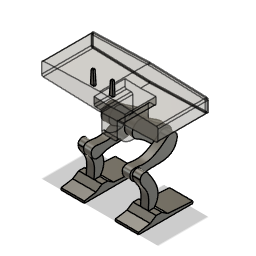
Mech v3 (Autodesk Fusion 360 design; units mm, degrees)
Autodesk Fusion 360 part; units mm, degrees
sketch "Esquisse1" plane through (0, 0, 0) normal (0, 0, 1) x (1, 0, 0)
  line L0 (-150, 33.8689) -> (-150, 61.1311)
  line L1 (-146.1333, 65.1289) -> (0, 70)
  line L2 (-146.1333, 29.8711) -> (0, 25)
  line L3 (146.1333, 65.1289) -> (0, 70)
  line L4 (150, 33.8689) -> (150, 61.1311)
  line L5 (146.1333, 29.8711) -> (0, 25)
  arc A0 (-146.1333, 65.1289) -> (-150, 61.1311) centre (-146, 61.1311) ccw
  arc A1 (-150, 33.8689) -> (-146.1333, 29.8711) centre (-146, 33.8689) ccw
  arc A2 (150, 61.1311) -> (146.1333, 65.1289) centre (146, 61.1311) ccw
  arc A3 (146.1333, 29.8711) -> (150, 33.8689) centre (146, 33.8689) ccw
  line L6 (146.0333, 62.1306) -> (0, 66.9983)
  line L7 (-146.0333, 62.1306) -> (0, 66.9983)
  arc A4 (-146.0333, 62.1306) -> (-147, 61.1311) centre (-146, 61.1311) ccw
  line L8 (-147, 33.8689) -> (-147, 61.1311)
  arc A5 (-147, 33.8689) -> (-146.0333, 32.8694) centre (-146, 33.8689) ccw
  line L9 (-146.0333, 32.8694) -> (0, 28.0017)
  line L10 (146.0333, 32.8694) -> (0, 28.0017)
  arc A6 (146.0333, 32.8694) -> (147, 33.8689) centre (146, 33.8689) ccw
  line L11 (147, 33.8689) -> (147, 61.1311)
  arc A7 (147, 61.1311) -> (146.0333, 62.1306) centre (146, 61.1311) ccw
  dimension "d3" = 4
  dimension "d4" = 4
  dimension "d5" = 4
  dimension "d6" = 4
  dimension "d7" = -3
  constraint tangent L0 A0
  constraint tangent L1 A0
  constraint tangent L2 A1
  constraint tangent L0 A1
  constraint tangent L3 A2
  constraint tangent L4 A2
  constraint tangent L5 A3
  constraint tangent L4 A3
  measures "d3" radius of A0
  measures "d4" radius of A1
  measures "d5" radius of A2
  measures "d6" radius of A3
extrude "Extrusion1" add sketch "Esquisse1" along normal blind 130 contours L0 L1 L2 L3 L4 L5 A0 A1 A2 A3 | L6 L7 A4 L8 A5 L9 L10 A6 L11 A7 makes body 1
extrude "Extrusion2" cut sketch "Esquisse1" along normal blind 5 contours L6 L7 A4 L8 A5 L9 L10 A6 L11 A7 bodies 1
move_body "Déplacer1" bodies 1 to x (1, 0, 0) y (0, 1, 0) z (0, 0, 1) at (0, 200, 0)
ref_plane "Plan de construction1" through (0, 225, 65) normal (0, 1, 0) x (0, 0, 1)
sketch "Esquisse2" plane through (0, 225, 0) normal (0, 1, 0) x (1, 0, 0)
  line L0 (40, -105) -> (-40, -105)
  line L1 (-40, -105) -> (-40, -25)
  line L2 (-40, -25) -> (40, -25)
  line L3 (40, -25) -> (40, -105)
  line L4 (146.1333, 0) -> (0, 0)
  dimension "d13" = 25
  constraint horizontal L0
  constraint vertical L1
  constraint horizontal L2
  constraint vertical L3
  measures "d13" distance of L2 L4
extrude "Extrusion3" cut sketch "Esquisse2" along normal blind 5 bodies 1
sketch "Esquisse3" plane through (0, 0, 105) normal (0, 0, -1) x (-1, 0, 0)
  line L0 (0, 225) -> (40, 226.3333)
  line L1 (40, 226.3333) -> (40, 230)
  line L2 (40, 230) -> (-40, 230)
  line L3 (-40, 230) -> (-40, 226.3333)
  line L4 (-40, 226.3333) -> (0, 225)
  line L5 (-40, 230) -> (40, 230)
  line L6 (40, 230) -> (40, 209)
  line L7 (36, 205) -> (24, 205)
  line L8 (20, 201) -> (20, 159)
  line L9 (16, 155) -> (-16, 155)
  line L10 (-20, 159) -> (-20, 201)
  line L11 (-24, 205) -> (-36, 205)
  line L12 (-40, 209) -> (-40, 230)
  arc A0 (-40, 209) -> (-36, 205) centre (-36, 209) ccw
  arc A1 (-20, 201) -> (-24, 205) centre (-24, 201) ccw
  arc A2 (-20, 159) -> (-16, 155) centre (-16, 159) ccw
  arc A3 (16, 155) -> (20, 159) centre (16, 159) ccw
  arc A4 (24, 205) -> (20, 201) centre (24, 201) ccw
  arc A5 (36, 205) -> (40, 209) centre (36, 209) ccw
  point P0 (20, 205)
  point P1 (20, 155)
  dimension "d16" = 50
  dimension "d17" = 4
  dimension "d18" = 4
  dimension "d19" = 4
  dimension "d20" = 4
  dimension "d21" = 4
  dimension "d22" = 4
  constraint coincident L2.end L3.start
  constraint coincident L1.end L2.start
  constraint perpendicular L5 L6
  constraint perpendicular L6 L7
  constraint perpendicular L7 L8
  constraint perpendicular L8 L9
  constraint perpendicular L9 L10
  constraint perpendicular L10 L11
  constraint perpendicular L5 L12
  constraint tangent L11 A0
  constraint tangent L12 A0
  constraint tangent L10 A1
  constraint tangent L11 A1
  constraint tangent L9 A2
  constraint tangent L10 A2
  constraint coincident P1 L9
  constraint coincident P1 L8
  constraint tangent L9 A3
  constraint tangent L8 A3
  constraint coincident P0 L8
  constraint coincident P0 L7
  constraint tangent L8 A4
  constraint tangent L7 A4
  constraint tangent L7 A5
  constraint tangent L6 A5
  measures "d16" distance of P0 P1
  measures "d17" radius of A0
  measures "d18" radius of A1
  measures "d19" radius of A2
  measures "d20" radius of A3
  measures "d21" radius of A4
  measures "d22" radius of A5
extrude "Extrusion4" add sketch "Esquisse3" along normal blind 80 bodies 1
sketch "Esquisse4" plane through (-20, 0, 0) normal (-1, 0, 0) x (0, 0, 1)
  line L0 (105, 159) -> (105, 201)
  line L1 (105, 201) -> (25, 201)
  line L2 (25, 201) -> (25, 159)
  line L3 (25, 159) -> (105, 159)
  line L4 (65, 205) -> (65, 155) construction
  line L5 (65, 155) -> (65, 205) construction
  arc A0 (25, 180) -> (105, 180) centre (65, 180) ccw
  line L6 (25, 180) -> (105, 180)
  dimension "d25" = 80
  constraint perpendicular L3 L4
  constraint midpoint L5 A0.centre
  constraint coincident L2 A0.start
  constraint coincident L0 A0.end
  constraint perpendicular L0 L6
  measures "d25" diameter of A0
extrude "Extrusion5" add sketch "Esquisse4" against normal blind 40 contours L3 A0 L6 | L3 A0 bodies 1
sketch "Esquisse5" plane through (-20, 0, 0) normal (-1, 0, 0) x (0, 0, 1)
  line L0 (25, 201) -> (25, 159)
  line L1 (25, 159) -> (30.9559, 159)
  arc A0 (30.9559, 159) -> (99.0441, 159) centre (65, 180) ccw
  line L2 (99.0441, 159) -> (105, 159)
  line L3 (105, 159) -> (105, 201)
  line L4 (105, 201) -> (25, 201)
  spline S0 degree 5 poles (50, 190) (48.5943, 188.5173) (45.7562, 185.6074) (41.4185, 181.4094) (35.4733, 176.1465) (27.7946, 170.1152) (19.9379, 164.5925) (12.0468, 159.4932) (4.3635, 154.6691) (-2.741, 149.8879) (-8.7472, 144.8223) (-13.1055, 139.1738) (-15.3557, 132.8001) (-15.2312, 125.8208) (-12.8105, 118.7889) (-8.4782, 112.5876) (-2.7614, 108.1375) (3.7842, 106.1866) (10.7306, 107.0074) (17.8284, 110.3413) (24.9477, 115.6146) (32.0463, 122.0851) (39.131, 129.0014) (46.216, 135.7855) (53.3085, 142.0733) (60.4134, 147.6486) (66.109, 151.4582) (70.3875, 153.9361) (73.2429, 155.4199) (74.6713, 156.1197) knots 0 0 0 0 0 0 0.04 0.08 0.12 0.16 0.2 0.24 0.28 0.32 0.36 0.4 0.44 0.48 0.52 0.56 0.6 0.64 0.68 0.72 0.76 0.8 0.84 0.88 0.92 0.96 1 1 1 1 1 1
  arc A1 (74.131, 155.8526) -> (49.3011, 189.2669) centre (65, 175) ccw
  point P0 (5, 155)
  point P1 (-15, 130)
  point P2 (0.8234, 107.4241)
  point P3 (35, 125)
  constraint coincident S0.start A1
  constraint coincident S0.end A1
  constraint coincident S0 A1.end
  constraint coincident S0 A1.start
extrude "Extrusion6" add sketch "Esquisse5" along normal blind 20 separate body contours L0 L1 A0 S0 A1 | L0 L1 A0 S0 makes body 2
sketch "Esquisse6" plane through (-40, 0, 0) normal (-1, 0, 0) x (0, 0, 1)
  spline S0 degree 5 poles (74.131, 155.8526) (74.2391, 155.9065) (74.3471, 155.9601) (74.4552, 156.0136) (74.5633, 156.0668) (74.6713, 156.1197) knots 0.996974 0.996974 0.996974 0.996974 0.996974 0.996974 1 1 1 1 1 1
  arc A0 (74.6713, 156.1197) -> (50, 190) centre (65, 175) ccw
  spline S1 degree 5 poles (50, 190) (49.8605, 189.8528) (49.7208, 189.7059) (49.5811, 189.5593) (49.4412, 189.413) (49.3011, 189.2669) knots 0 0 0 0 0 0 0.00397 0.00397 0.00397 0.00397 0.00397 0.00397
  spline S2 degree 5 poles (49.3011, 189.2669) (48.0302, 187.9413) (45.3253, 185.1916) (41.1233, 181.1485) (35.3209, 176.0267) (27.7946, 170.1152) (19.9379, 164.5925) (12.0468, 159.4932) (4.3635, 154.6691) (-2.741, 149.8879) (-8.7472, 144.8223) (-13.1055, 139.1738) (-15.3557, 132.8001) (-15.2312, 125.8208) (-12.8105, 118.7889) (-8.4782, 112.5876) (-2.7614, 108.1375) (3.7842, 106.1866) (10.7306, 107.0074) (17.8284, 110.3413) (24.9477, 115.6146) (32.0463, 122.0851) (39.131, 129.0014) (46.216, 135.7855) (53.3085, 142.0733) (60.3059, 147.5642) (65.8935, 151.3139) (70.0638, 153.7479) (72.8109, 155.1939) (74.131, 155.8526) knots 0.00397 0.00397 0.00397 0.00397 0.00397 0.00397 0.04 0.08 0.12 0.16 0.2 0.24 0.28 0.32 0.36 0.4 0.44 0.48 0.52 0.56 0.6 0.64 0.68 0.72 0.76 0.8 0.84 0.88 0.92 0.96 0.996974 0.996974 0.996974 0.996974 0.996974 0.996974
  spline S3 degree 5 poles (-8.5063, 123.5236) (-8.1226, 121.791) (-7.2435, 118.4579) (-5.5903, 113.854) (-2.7158, 108.5079) (1.9828, 103.1375) (7.7462, 99.0459) (14.4865, 96.1594) (22.0545, 94.3508) (30.2168, 93.4202) (38.6554, 93.0927) (47.0224, 93.0622) (54.9848, 93.0257) (62.2732, 92.7217) (68.7283, 91.9664) (74.3503, 90.6921) (79.3449, 88.984) (84.0154, 87.0599) (88.6532, 85.2541) (93.439, 83.9929) (98.3134, 83.7935) (103.0122, 85.1344) (107.1615, 88.274) (110.3514, 93.094) (112.2218, 98.9085) (112.4972, 104.726) (111.0241, 109.5548) (107.8019, 112.6688) (103.0306, 113.9507) (97.0589, 113.7856) (90.3019, 112.823) (83.1723, 111.7929) (75.9995, 111.2806) (68.9759, 111.5793) (62.1958, 112.7798) (55.6779, 114.8205) (49.3948, 117.5544) (43.2975, 120.8045) (37.3462, 124.4325) (31.5155, 128.3494) (25.7893, 132.4999) (21.2856, 135.9852) (17.95, 138.6875) (15.745, 140.5283) (14.6471, 141.4585) knots 0 0 0 0 0 0 0.025 0.05 0.075 0.1 0.125 0.15 0.175 0.2 0.225 0.25 0.275 0.3 0.325 0.35 0.375 0.4 0.425 0.45 0.475 0.5 0.525 0.55 0.575 0.6 0.625 0.65 0.675 0.7 0.725 0.75 0.775 0.8 0.825 0.85 0.875 0.9 0.925 0.95 0.975 1 1 1 1 1 1
  arc A1 (14.7156, 141.4005) -> (-8.5063, 123.5236) centre (5, 130) ccw
  point P0 (20, 95)
  point P1 (68.4132, 91.856)
  point P2 (90, 85)
  point P3 (107.1929, 88.9905)
  point P4 (110, 110)
  point P5 (84.842, 112.1055)
  point P6 (47.5906, 118.6006)
  constraint coincident S3.end A1
  constraint coincident S3 A1.start
extrude "Extrusion7" add sketch "Esquisse6" along normal blind 20 contours S2 S3 | S2 S3 A1 bodies 2
sketch "Esquisse7" plane through (-60, 0, 0) normal (-1, 0, 0) x (0, 0, 1)
  line L0 (14.7156, 141.4005) -> (14.6471, 141.4585)
  arc A0 (14.6471, 141.4585) -> (-8.5063, 123.5236) centre (5, 130) ccw
  spline S0 degree 5 poles (-8.5063, 123.5236) (-8.1226, 121.791) (-7.2435, 118.4579) (-5.5903, 113.854) (-2.7158, 108.5079) (1.9828, 103.1375) (7.7462, 99.0459) (14.4865, 96.1594) (22.0545, 94.3508) (30.2168, 93.4202) (38.6554, 93.0927) (47.0224, 93.0622) (54.9848, 93.0257) (62.2732, 92.7217) (68.7283, 91.9664) (74.3503, 90.6921) (79.3449, 88.984) (84.0154, 87.0599) (88.6532, 85.2541) (93.439, 83.9929) (98.3134, 83.7935) (103.0122, 85.1344) (107.1615, 88.274) (110.3514, 93.094) (112.2218, 98.9085) (112.4972, 104.726) (111.0241, 109.5548) (107.8019, 112.6688) (103.0306, 113.9507) (97.0589, 113.7856) (90.3019, 112.823) (83.1723, 111.7929) (75.9995, 111.2806) (68.9759, 111.5793) (62.1958, 112.7798) (55.6779, 114.8205) (49.3948, 117.5544) (43.2975, 120.8045) (37.3462, 124.4325) (31.5155, 128.3494) (25.8036, 132.4895) (21.3137, 135.9634) (17.9916, 138.6538) (15.7999, 140.4824) (14.7156, 141.4005) knots 0 0 0 0 0 0 0.025 0.05 0.075 0.1 0.125 0.15 0.175 0.2 0.225 0.25 0.275 0.3 0.325 0.35 0.375 0.4 0.425 0.45 0.475 0.5 0.525 0.55 0.575 0.6 0.625 0.65 0.675 0.7 0.725 0.75 0.775 0.8 0.825 0.85 0.875 0.9 0.925 0.95 0.975 0.999688 0.999688 0.999688 0.999688 0.999688 0.999688
  spline S1 degree 5 poles (84.4841, 103.2274) (83.0085, 101.166) (80.154, 97.0756) (76.1623, 91.0374) (71.4299, 83.1848) (66.5704, 73.724) (62.8807, 64.6564) (60.4933, 56.0265) (59.5296, 47.8752) (60.0385, 40.2189) (61.9589, 33.037) (64.5542, 27.6473) (67.0622, 23.7939) (68.9798, 21.3075) (70, 20.0849) knots 0 0 0 0 0 0 0.1 0.2 0.3 0.4 0.5 0.6 0.7 0.8 0.9 1 1 1 1 1 1
  spline S2 degree 5 poles (106, 100) (106, 98.7107) (105.838, 96.1843) (105.1087, 92.5515) (103.2345, 87.99) (99.8024, 82.5801) (95.8269, 77.2362) (91.8872, 71.7356) (88.4972, 65.9101) (86.0067, 59.6978) (84.4968, 53.1998) (83.856, 46.6287) (83.8501, 40.2612) (84.1893, 34.3904) (84.5883, 29.2814) (84.8343, 25.1174) (84.8325, 22.5956) (84.7064, 21.1632) (84.5674, 20.4106) (84.4841, 20.0849) knots 0 0 0 0 0 0 0.066667 0.133333 0.2 0.266667 0.333333 0.4 0.466667 0.533333 0.6 0.666667 0.733333 0.8 0.866667 0.933333 1 1 1 1 1 1
  line L1 (70, 20.0849) -> (55, 10)
  line L2 (100, 10) -> (84.4841, 20.0849)
  line L3 (55, 10) -> (-10, 5)
  line L4 (-10, 5) -> (-10, 0)
  line L5 (-10, 0) -> (130, 0)
  line L6 (130, 0) -> (130, 5)
  line L7 (130, 5) -> (100, 10)
  arc A1 (106, 100) -> (84.4841, 103.2274) centre (95, 100) ccw
  line L8 (70, 20.0849) -> (84.4841, 20.0849)
  point P0 (60, 50)
  point P1 (88.7009, 65.7756)
  point P2 (84.4841, 30.4969)
  dimension "d32" = 22
  constraint tangent S2 A1
  constraint perpendicular L4 L5
  constraint horizontal L8
  measures "d32" diameter of A1
extrude "Extrusion8" add sketch "Esquisse7" along normal blind 20 contours S0 S1 S2 L8 | S0 S1 S2 A1 bodies 2
extrude "Extrusion9" add sketch "Esquisse7" along normal blind 40 and the other way blind 20 contours L1 L2 L3 L4 L5 L6 L7 L8 bodies 2
mirror "Symétrie miroir1" about plane through (0, 0, 0) normal (1, 0, 0) of bodies 2 makes body 3
ref_plane "Plan de construction2" through (0, 247.5, 125) normal (0, 0, 1) x (1, 0, 0)
sketch "Esquisse8" plane through (0, 0, 125) normal (0, 0, 1) x (1, 0, 0)
  line L0 (-25, 269) -> (-19.7782, 269)
  line L1 (-19.7782, 269) -> (-22.3891, 304.2057)
  line L2 (-22.3891, 304.2057) -> (-27.3754, 303.8359)
  line L3 (-27.3754, 303.8359) -> (-29, 269)
  line L4 (-29, 269) -> (-25, 269)
  line L5 (0, 314) -> (0, 260) construction
  line L6 (22.3891, 304.2057) -> (27.3754, 303.8359)
  line L7 (27.3754, 303.8359) -> (29, 269)
  line L8 (19.7782, 269) -> (22.3891, 304.2057)
  line L9 (25, 269) -> (19.7782, 269)
  line L10 (29, 269) -> (25, 269)
  dimension "d42" = 5
  constraint horizontal L0
  constraint perpendicular L1 L2
  constraint parallel L0 L4
  constraint symmetric L0.start L5 L9.start
  constraint symmetric L0.end L5 L8.start
  constraint symmetric L1.end L5 L6.start
  constraint symmetric L2.end L5 L6.end
  constraint symmetric L3.end L5 L7.end
  measures "d42" distance of L1.end L2.end
extrude "Extrusion10" add sketch "Esquisse8" against normal blind 5 separate body makes body 4 at (25.3845, 280.612, 125) makes body 5 at (-25.3845, 280.612, 125)
